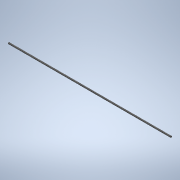
# Autodesk Inventor part: IISRD_CFR_4x5_556mm
Saved by Autodesk Inventor 2021 (Build 250183000, 183)
## iProperties
Created: 2020-10-19
Part Number: IISRD_CFR_4x5_556mm
Material: CFRP
Document SubType Name: Modeling
Designer: Kanenas
Mass: 6.57082 g
Surface Area: 159.991 cm^2
Volume: 4.59498 cm^3
Density: 1.43 g/cm^3
Appearance: Carbon Fiber
Author: Kanenas
Autodesk Inventor part; units mm, degrees
ref_plane "YZ Plane" through (0, 0, 0) normal (1, 0, 0) x (0, 1, 0)
ref_plane "XZ Plane" through (0, 0, 0) normal (0, 1, 0) x (-1, 0, 0)
ref_plane "XY Plane" through (0, 0, 0) normal (0, 0, 1) x (1, 0, 0)
sketch "Sketch1" plane through (0, 0, 0) normal (1, 0, 0) x (0, 1, 0)
  circle A0 centre (0, 0) radius 2
  circle A1 centre (0, 0) radius 2.575
  dimension "d0" = 4
  dimension "d1" = 5.15
  constraints: 2 centre point, 2 coincident
  measures "d0" diameter of A0
  measures "d1" diameter of A1
extrude "Extrusion1" add sketch "Sketch1" along normal blind 556
body "Solid1"
